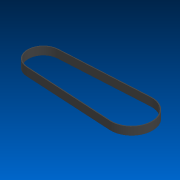
# Autodesk Inventor part: 110T x 9mm Wide Timing Belt (GT2 3mm) (217-5890)
Saved by Autodesk Inventor 2022.2 (Build 262287000, 287)
## iProperties
Created: 2022-01-07
Part Number: 110T x 9mm Wide Timing Belt (GT2 3mm) (217-5890)
Material: Rubber, Black
Document SubType Name: Modeling
Designer: omard
Density: 0.93 g/cm^3
Appearance: Rubber - Black
Author: omard
Autodesk Inventor part; units mm, degrees
ref_plane "YZ Plane" through (0, 0, 0) normal (1, 0, 0) x (0, 1, 0)
ref_plane "XZ Plane" through (0, 0, 0) normal (0, 1, 0) x (-1, 0, 0)
ref_plane "XY Plane" through (0, 0, 0) normal (0, 0, 1) x (1, 0, 0)
sketch "Sketch1" plane through (0, 0, 0) normal (0, 1, 0) x (-1, 0, 0)
  arc A0 (102.0812, -17.1554) -> (102.0812, 17.1554) centre (101.1056, 0) ccw
  arc A1 (1.3015, 22.8865) -> (1.3015, -22.8865) centre (0, 0) ccw
  line L0 (102.0812, -17.1554) -> (1.3015, -22.8865)
  line L1 (102.0812, 17.1554) -> (1.3015, 22.8865)
  line L2 (1.3583, -23.8849) -> (102.138, -18.1538)
  arc A2 (102.138, -18.1538) -> (102.138, 18.1538) centre (101.1056, 0) ccw
  line L3 (102.138, 18.1538) -> (1.3583, 23.8849)
  arc A3 (1.3583, 23.8849) -> (1.3583, -23.8849) centre (0, 0) ccw
  dimension "d0" = 101.1056
  dimension "d1" = 34.3662
  dimension "d2" = 45.847
  dimension "d6" = 1
  constraints: 8 end point, 8 point on circle, 4 centre point, 4 tangent, 1 coincident, 1 horizontal alignment, 3 other
  measures "d0" distance of point (0, 0) A0.centre
  measures "d1" diameter of A0
  measures "d2" diameter of A1
  measures "d6" distance between parallel lines of L0 L2
extrude "Extrusion1" add sketch "Sketch1" along normal mid plane 9
body "Solid1"
